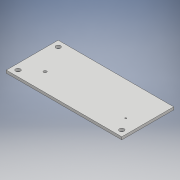
# Autodesk Inventor part: ShieldBare
Saved by Autodesk Inventor 2017 (Build 210142000, 142)
## iProperties
Created: 2017-06-22
Part Number: ShieldBare
Material: Generic
Document SubType Name: Modeling
Designer: P. Baesso
Density: 1 g/cm^3
Appearance: Default
Author: P. Baesso
Autodesk Inventor part; units mm, degrees
ref_plane "YZ Plane" through (0, 0, 0) normal (1, 0, 0) x (0, 1, 0)
ref_plane "XZ Plane" through (0, 0, 0) normal (0, 1, 0) x (-1, 0, 0)
ref_plane "XY Plane" through (0, 0, 0) normal (0, 0, 1) x (1, 0, 0)
sketch "Sketch1" plane through (0, 0, 0) normal (0, 0, 1) x (1, 0, 0)
  line L0 (0, -53) -> (79, -53) projected
  line L1 (82, -50) -> (82, 0) projected
  circle A0 centre (78.5, -49.5) radius 1.375 projected
  circle A1 centre (20.5, -49.5) radius 1.375 projected
  line L2 (35.3891, -15.1062) -> (35.3891, -19.5) projected
  line L3 (35.3891, -19.5) -> (38.2391, -19.5) projected
  line L4 (38.2391, -19.5) -> (38.2391, -16.9) projected
  line L5 (38.2391, -16.9) -> (36.6891, -16.9) projected
  line L6 (36.6891, -16.9) -> (36.6891, -0.1) projected
  line L7 (36.6891, -0.1) -> (38.2391, -0.1) projected
  line L8 (38.2391, -0.1) -> (38.2391, 2.5) projected
  line L9 (38.2391, 2.5) -> (35.3891, 2.5) projected
  line L10 (35.3891, 2.5) -> (35.3891, -1.8938) projected
  line L11 (35.3891, -1.8938) -> (34.3391, -2.5) projected
  line L12 (34.3391, -2.5) -> (34.3391, -14.5) projected
  line L13 (34.3391, -14.5) -> (35.3891, -15.1062) projected
  line L14 (12.09, -50.25) -> (12.09, -37.75) projected
  circle A2 centre (25.37, -48.23) radius 0.9016 projected
  circle A3 centre (25.37, -50.77) radius 0.9016 projected
  circle A4 centre (73.63, -50.77) radius 0.9016 projected
  circle A5 centre (73.63, -48.23) radius 0.474 projected
  line L15 (13, -59) -> (82, -59)
  line L16 (82, -59) -> (82, -28)
  line L17 (82, -28) -> (13, -28)
  line L18 (13, -28) -> (13, -59)
  circle A6 centre (16.5, -55.5) radius 1.375
  circle A7 centre (16.5, -31.5) radius 1.375
  circle A8 centre (78.5, -55.5) radius 1.375
  point P0 (0, 0)
  dimension "d0" = 69
  dimension "d1" = 6
  dimension "d2" = 25
  dimension "d3" = 2.75
  dimension "d4" = 3.5
  dimension "d5" = 3.5
  dimension "d6" = 2.75
  dimension "d7" = 3.5
  dimension "d8" = 3.5
  dimension "d9" = 2.75
  dimension "d10" = 3.5
  dimension "d11" = 3.5
  constraints: 8 end point, 3 centre point, 2 parallel, 1 horizontal, 1 perpendicular, 1 point on line
  measures "d0" distance of L15.start L15.end
  measures "d1" distance between parallel lines of L15 L0
  measures "d2" distance between parallel lines of L17 L0
  measures "d3" diameter of A6
  measures "d4" distance from line of L15 A6.centre
  measures "d5" distance from line of L18 A6.centre
  measures "d6" diameter of A7
  measures "d7" distance from line of L18 A7.centre
  measures "d8" distance from line of L17 A7.centre
  measures "d9" diameter of A8
  measures "d10" distance from line of L16 A8.centre
  measures "d11" distance from line of A8.centre L15
extrude "Extrusion1" add sketch "Sketch1" along normal blind 1.6 contours L16 L15 L18 L17 L1 | A0 | A1 | A3 | A4
body "Solid1"
